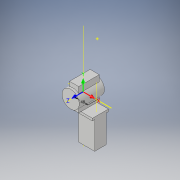
# Autodesk Inventor part: link_3
Saved by Autodesk Inventor 2019 (Build 230136000, 136)
## iProperties
Created: 2020-08-30
Part Number: link_3
Material: Generic
Document SubType Name: Modeling
Designer: Daniel
Density: 1 g/cm^3
Appearance: Default
Author: Daniel
Autodesk Inventor part; units mm, degrees
ref_plane "YZ Plane" through (0, 0, 0) normal (1, 0, 0) x (0, 1, 0)
ref_plane "XY Plane" through (0, 0, 0) normal (0, 0, 1) x (1, 0, 0)
sketch "Sketch1" plane through (0, 0, 0) normal (0, 0, 1) x (1, 0, 0)
  circle A0 centre (0, 0) radius 30
  dimension "d0" = 60
  constraints: 1 centre point, 1 coincident
  measures "d0" diameter of A0
extrude "Extrusion1" add sketch "Sketch1" along normal mid plane 88
sketch "Sketch2" plane through (0, 0, 0) normal (0, 1, 0) x (-1, 0, 0)
  line L0 (51.4648, 0) -> (-98.7887, 0) projected
  line L1 (0, -61.6) -> (0, 61.6) projected
  point P0 (0, 0)
  point P1 (-48, 0)
  dimension "d11" = 48
  constraints: 1 point on line
  measures "d11" distance from line of L1 point (-48, 0)
ref_plane "Work Plane1" through (0, -36, 0) normal (0, 1, 0) x (-1, 0, 0)
sketch "Sketch3" plane through (0, -36, 0) normal (0, 1, 0) x (-1, 0, 0)
  line L0 (12, -28) -> (-60, -28)
  line L1 (-60, -28) -> (-60, 28)
  line L2 (-60, 28) -> (12, 28)
  line L3 (12, 28) -> (12, -28)
  line L4 (12, -28) -> (-60, 28) construction
  line L5 (-60, -28) -> (12, 28) construction
  line L6 (47.0012, 0) -> (-72.0071, 0) projected
  point P0 (0, 0)
  point P1 (-24, 0)
  point P2 (-24, 0)
  point P3 (-48, 0)
  dimension "d13" = 12
  dimension "d14" = 56
  dimension "d15" = 60
  constraints: 12 end point, 3 midpoint, 2 parallel, 1 horizontal, 1 perpendicular, 1 point on line
  measures "d13" distance from line of L1 point (-48, 0)
  measures "d14" distance between parallel lines of L0 L2
  measures "d15" distance from line of L3 point (-48, 0)
extrude "Extrusion2" add sketch "Sketch3" against normal blind 8
sketch "Sketch4" plane through (0, -36, 0) normal (0, 1, 0) x (1, 0, 0)
  line L0 (-12, -36) -> (20, -36)
  line L1 (20, -36) -> (20, 36)
  line L2 (20, 36) -> (-12, 36)
  line L3 (-12, 36) -> (-12, -36)
  line L4 (-12, -36) -> (20, 36) construction
  line L5 (20, -36) -> (-12, 36) construction
  line L6 (-48, 0) -> (78, 0) projected
  line L7 (-12, -28) -> (-12, 28) projected
  line L8 (60, -28) -> (-12, -28) projected
  point P0 (0, 0)
  point P1 (4, 0)
  point P2 (4, 0)
  dimension "d18" = 32
  dimension "d19" = 8
  constraints: 12 end point, 3 midpoint, 2 parallel, 1 collinear, 1 horizontal, 1 perpendicular, 1 point on line
  measures "d18" distance between parallel lines of L7 L1
  measures "d19" distance between parallel lines of L8 L0
extrude "Extrusion3" add sketch "Sketch4" along normal blind 80
sketch "Sketch5" plane through (0, -44, 0) normal (0, -1, 0) x (1, 0, 0)
  line L0 (60, -28) -> (60, 28) projected
  line L1 (4, 20) -> (60, 20)
  line L2 (60, 20) -> (60, -20)
  line L3 (60, -20) -> (4, -20)
  line L4 (4, -20) -> (4, 20)
  line L5 (4, 20) -> (60, -20) construction
  line L6 (60, 20) -> (4, -20) construction
  line L7 (-48, 0) -> (78, 0) projected
  point P0 (0, 0)
  point P1 (32, 0)
  point P2 (32, 0)
  dimension "d22" = 40
  dimension "d23" = 56
  constraints: 12 end point, 3 midpoint, 2 parallel, 2 point on line, 1 horizontal, 1 perpendicular
  measures "d22" distance of L3.end L1.start
  measures "d23" distance between parallel lines of L0 L4
extrude "Extrusion4" add sketch "Sketch5" along normal blind 96
ref_plane "Work Plane2" through (0, 184, 0) normal (0, 1, 0) x (-1, 0, 0)
ref_plane "UCS3: YZ Plane" through (0, 0, 0) normal (1, 0, 0) x (0, 1, 0)
ref_plane "UCS3: XZ Plane" through (0, 0, 0) normal (0, 1, 0) x (0, 0, 1)
ref_plane "UCS3: XY Plane" through (0, 0, 0) normal (0, 0, 1) x (1, 0, 0)
body "Solid1"
